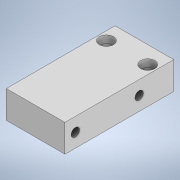
# Autodesk Inventor part: 本体
Saved by Autodesk Inventor 2021 (Build 250183000, 183)
## iProperties
Created: 2021-09-24
Part Number: 本体
Material: 一般
Document SubType Name: Modeling
Designer: tomat
Density: 1 g/cm^3
Appearance: 既定
Author: tomat
Autodesk Inventor part; units mm, degrees
ref_plane "YZ Plane" through (0, 0, 0) normal (1, 0, 0) x (0, 1, 0)
ref_plane "XZ Plane" through (0, 0, 0) normal (0, 1, 0) x (-1, 0, 0)
ref_plane "XY Plane" through (0, 0, 0) normal (0, 0, 1) x (1, 0, 0)
sketch "スケッチ1" plane through (0, 0, 0) normal (0, 1, 0) x (-1, 0, 0)
  line L0 (0, 0) -> (17, 0)
  line L1 (17, 0) -> (17, -31.5)
  line L2 (17, -31.5) -> (0, -31.5)
  line L3 (0, -31.5) -> (0, 0)
  dimension "d0" = 17
  dimension "d1" = 31.5
  constraints: 8 end point, 2 parallel, 1 horizontal, 1 perpendicular
  measures "d0" distance of L1.end L2.end
  measures "d1" distance of L0.end L1.end
extrude "押し出し1" add sketch "スケッチ1" along normal blind 8
sketch "スケッチ2" plane through (0, 0, 0) normal (1, 0, 0) x (0, 0, -1)
  line L0 (31.5, 0) -> (31.5, 8) projected
  line L1 (0, 0) -> (31.5, 0) projected
  point P0 (21.5, 4)
  point P1 (3, 4)
  dimension "d4" = 10
  dimension "d5" = 18.5
  dimension "d6" = 4
  dimension "d7" = 4
  measures "d4" distance from line of L0 point (21.5, 4)
  measures "d5" distance of point (21.5, 4) point (3, 4)
  measures "d6" distance from line of L1 point (21.5, 4)
  measures "d7" distance from line of L1 point (3, 4)
hole "穴1" at (0, 4, -21.5) at (0, 4, -3) direction (-1, 0, 0) diameter 2.459 depth 6 tip angle 118 thread size "M3x0.5" class "6H" standard "ISO Metric profile"
sketch "スケッチ3" plane through (0, 0, -31.5) normal (0, 0, -1) x (-1, 0, 0)
  line L0 (0, 0) -> (17, 0) projected
  line L1 (0, 0) -> (0, 8) projected
  point P0 (2.5, 4)
  point P1 (14.5, 4)
  dimension "d15" = 4
  dimension "d16" = 4
  dimension "d17" = 2.5
  dimension "d18" = 12
  measures "d15" distance from line of L0 point (2.5, 4)
  measures "d16" distance from line of L0 point (14.5, 4)
  measures "d17" distance from line of L1 point (2.5, 4)
  measures "d18" distance of point (14.5, 4) point (2.5, 4)
hole "穴2" at (-2.5, 4, -31.5) at (-14.5, 4, -31.5) direction (0, 0, 1) diameter 2.459 depth 4 tip angle 118 thread size "M3x0.5" class "6H" standard "ISO Metric profile"
sketch "スケッチ4" plane through (0, 8, 0) normal (0, 1, 0) x (1, 0, 0)
  line L0 (0, 31.5) -> (-17, 31.5) projected
  line L1 (0, 0) -> (0, 31.5) projected
  point P0 (-2.5, 26.5)
  point P1 (-14.5, 26.5)
  dimension "d26" = 5
  dimension "d27" = 5
  dimension "d28" = 2.5
  dimension "d29" = 12
  measures "d26" distance from line of L0 point (-2.5, 26.5)
  measures "d27" distance from line of L0 point (-14.5, 26.5)
  measures "d28" distance from line of L1 point (-2.5, 26.5)
  measures "d29" distance of point (-2.5, 26.5) point (-14.5, 26.5)
hole "穴3" at (-2.5, 8, -26.5) at (-14.5, 8, -26.5) direction (0, -1, 0) diameter 4.1 depth 2.2 tip angle 118
sketch "スケッチ5" plane through (0, 8, 0) normal (0, 1, 0) x (1, 0, 0)
  circle A0 centre (-2.5, 26.5) radius 2.05 projected
  circle A1 centre (-14.5, 26.5) radius 2.05 projected
  point P0 (0, 0)
  constraints: 2 coincident
hole "穴4" at (-2.5, 8, -26.5) at (-14.5, 8, -26.5) at (-2.5, 8, -26.5) at (-14.5, 8, -26.5) direction (0, -1, 0) diameter 2.2 end through all
sketch "スケッチ6" plane through (0, 0, 0) normal (0, -1, 0) x (1, 0, 0)
  circle A0 centre (-14.5, -26.5) radius 2.05 projected
  arc A1 (-2.4721, -27.5996) -> (-2.5279, -27.5996) centre (-2.5, -26.5) ccw projected
  point P0 (0, 0)
  constraints: 2 coincident
hole "穴5" at (-14.5, 0, -26.5) at (-2.5, 0, -26.5) direction (0, 1, 0) diameter 4.1 depth 2.2 tip angle 118
sketch "スケッチ7" plane through (0, 0, -31.5) normal (0, 0, -1) x (-1, 0, 0)
  line L0 (0, 0) -> (17, 0) projected
  line L1 (17, 0) -> (17, 8) projected
  point P0 (8.5, 4)
  dimension "d51" = 4
  dimension "d52" = 8.5
  measures "d51" distance from line of L0 point (8.5, 4)
  measures "d52" distance from line of L1 point (8.5, 4)
hole "穴6" at (-8.5, 4, -31.5) direction (0, 0, 1) diameter 3 depth 15 tip angle 118
